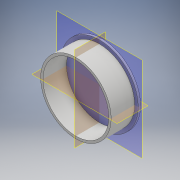
# Autodesk Inventor part: Крышка и батарейный отсек
Saved by Autodesk Inventor 2017 (Build 210142000, 142)
## iProperties
Part Number: Крышка и батарейный отсек
Material: Типовые
Document SubType Name: Modeling
Designer: Arseny Radushin
Density: 1 g/cm^3
Appearance: По умолчанию
Author: Arseny Radushin
Autodesk Inventor part; units mm, degrees
sketch "Эскиз5" plane through (0, 0, 0) normal (0, 1, 0) x (-1, 0, 0)
  circle A0 centre (0, 0) radius 16.5
  dimension "d12" = 33
  constraints: 1 centre point, 1 coincident
  measures "d12" diameter of A0
extrude "Выдавливание4" add sketch "Эскиз5" along normal blind 1
sketch "Эскиз7" plane through (0, 1, 0) normal (0, 1, 0) x (1, 0, 0)
  circle A0 centre (0, 0) radius 16
  circle A1 centre (0, 0) radius 16.5 projected
  arc A2 (-0.5, 14.9917) -> (-0.5354, 14.9904) centre (0, 0) ccw
  line L0 (0.5, -14) -> (-0.5, -14)
  line L1 (-0.5, 14) -> (0.5, 14)
  line L2 (0.5, -14) -> (-0.5, 14) construction
  line L3 (-0.5, -14) -> (0.5, 14) construction
  line L4 (-0.5, -14) -> (0.5, -14)
  line L5 (0.5, -14) -> (0.5, -15.4866)
  line L6 (0.5, -15.4866) -> (-0.5, -15.4866)
  line L7 (-0.5, -15.4866) -> (-0.5, -14)
  line L8 (0.5, 14) -> (-0.5, 14)
  line L9 (-0.5, 14) -> (-0.5, 15.7701)
  line L10 (-0.5, 15.7701) -> (0.5, 15.7701)
  line L11 (0.5, 15.7701) -> (0.5, 14)
  arc A3 (0.5, -14.9917) -> (0.5354, 14.9904) centre (0, 0) ccw
  arc A4 (0.5354, 14.9904) -> (0.5, 14.9917) centre (0, 0) ccw
  arc A5 (-0.5354, 14.9904) -> (-0.5, -14.9917) centre (0, 0) ccw
  dimension "d17" = 1
  dimension "d18" = 28
  dimension "d19" = 32
  dimension "d21" = 2.045
  dimension "d22" = 177.955
  dimension "d23" = 0
  dimension "d24" = 1.7701
  dimension "d25" = 31.2568
  dimension "d26" = 0.5
  dimension "d27" = 15.7701
  dimension "d30" = 15
  dimension "d31" = 15
  constraints: 24 end point, 8 point on circle, 7 point on line, 5 centre point, 5 parallel, 3 horizontal, 2 midpoint, 2 perpendicular, 1 coincident
  measures "d17" distance of L1.start L1.end
  measures "d18" distance of L0.end L1.start
  measures "d19" diameter of A0
  measures "d21" angle of L11 L2
  measures "d22" angle of L11 L3
  measures "d23" distance between parallel lines of L11 L5
  measures "d24" distance between parallel lines of L10 L1
  measures "d25" distance between parallel lines of L10 L6
  measures "d26" distance from line of A0.centre L11
  measures "d27" distance from line of A0.centre L10
  measures "d30" radius of A4
  measures "d31" radius of A2
extrude "Выдавливание6" add sketch "Эскиз7" along normal blind 1 contours L9 L1 L11 A4 A3 L5 L0 L7 A5 A2
sketch "Эскиз9" plane through (0, 0, 0) normal (0, -1, 0) x (1, 0, 0)
  circle A0 centre (0, 0) radius 15
  circle A1 centre (0, 0) radius 14
  dimension "d41" = 30
  dimension "d42" = 28
  constraints: 2 centre point, 2 coincident
  measures "d41" diameter of A0
  measures "d42" diameter of A1
extrude "Выдавливание8" add sketch "Эскиз9" along normal blind 10
